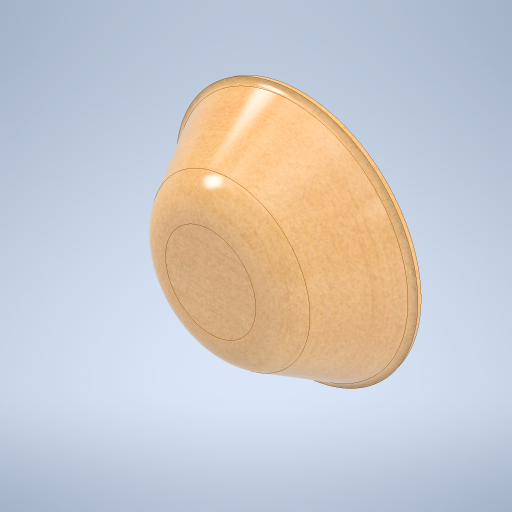
# Autodesk Inventor part: Bol
Saved by Autodesk Inventor 2024 (Build 280153000, 153)
## iProperties
Created: 2024-03-22
Part Number: Bol
Material: Stahl, galvanisiert
Document SubType Name: Modeling
Designer: ffogue
Density: 7.85 g/cm^3
Appearance: Gelbkiefer - gebeizt - dunkel - mittlerer Glanz
Author: ffogue
Autodesk Inventor part; units mm, degrees
ref_plane "YZ Plane" through (0, 0, 0) normal (1, 0, 0) x (0, 1, 0)
ref_plane "XZ Plane" through (0, 0, 0) normal (0, 1, 0) x (-1, 0, 0)
ref_plane "XY Plane" through (0, 0, 0) normal (0, 0, 1) x (1, 0, 0)
sketch "Skizze1" plane through (0, 0, 0) normal (0, 0, 1) x (1, 0, 0)
  line L0 (0, 0) -> (0, 393.6564) construction
  line L1 (0, 0) -> (60, 0)
  line L2 (60, 0) -> (101.7513, 72.3153)
  line L3 (106.188, 80) -> (0, 80)
  arc A0 (106.6863, 76.0631) -> (101.7513, 72.3153) centre (108.6795, 68.3153) ccw
  arc A1 (106.6863, 76.0631) -> (106.188, 80) centre (106.188, 78) ccw
  line L4 (0, 0) -> (0, 80)
  dimension "d1" = 30
  dimension "d2" = 80
  dimension "d3" = 120
  dimension "d4" = 2
  dimension "d5" = 8
  constraints: 10 end point, 4 point on circle, 3 tangent, 2 centre point, 2 point on line, 1 collinear, 1 horizontal, 1 perpendicular, 1 vertical
  measures "d1" angle of L0 L2
  measures "d2" distance between parallel lines of L1 L3
  measures "d3" diameter of L1.end L0
  measures "d4" radius of A1
  measures "d5" radius of A0
revolve "Umdrehung1" add sketch "Skizze1" angle 360 about axis through (0, 0, 0) along (0, 1, 0)
fillet "Rundung2" radius 35 1 edges at (-60, 0, 0)
shell "Wandung5" thickness 4 removed faces 2 at (6.6674, 80, -32.0854) at (-108.0747, 77.9307, -4.9241)
